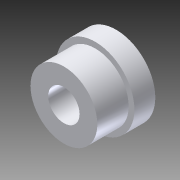
# Autodesk Inventor part: upper_cap
Saved by Autodesk Inventor 2011 SP2 (Build 150309200, 309)
## iProperties
Created: 2013-09-16
Part Number: upper_cap
Document SubType Name: Modeling
Designer: sungwook
Density: 1.42 g/cm^3
Material: Acetal Resin, White
Mass: 0.0319958 g
Surface Area: 0.659143 cm^2
Volume: 0.0225323 cm^3
Author: sungwook
Autodesk Inventor part; units mm, degrees
ref_plane "YZ Plane" through (0, 0, 0) normal (1, 0, 0) x (0, 1, 0)
ref_plane "XZ Plane" through (0, 0, 0) normal (0, 1, 0) x (-1, 0, 0)
ref_plane "XY Plane" through (0, 0, 0) normal (0, 0, 1) x (1, 0, 0)
sketch "Sketch1" plane through (0, 0, 0) normal (0, 0, 1) x (1, 0, 0)
  circle A0 centre (0, 0) radius 1.905
  dimension "d0" = 3.81
  constraints: 1 centre point, 1 coincident
  measures "d0" diameter of A0
extrude "Extrusion1" add sketch "Sketch1" along normal blind 1.016
sketch "Sketch2" plane through (0, 0, 1.016) normal (0, 0, 1) x (1, 0, 0)
  circle A0 centre (0, 0) radius 1.905 projected
  circle A1 centre (0, 0) radius 1.6256
  dimension "d3" = 3.2512
  constraints: 1 centre point, 1 coincident
  measures "d3" diameter of A1
extrude "Extrusion2" add sketch "Sketch2" along normal blind 1.524 contours A1
sketch "Sketch3" plane through (0, 0, 0) normal (0, 0, -1) x (-1, 0, 0)
  circle A0 centre (0, 0) radius 1.905 projected
hole "Hole1" at (0, 0, 0) direction (0, 0, 1) diameter 1.524 end through all
body "Solid1"
